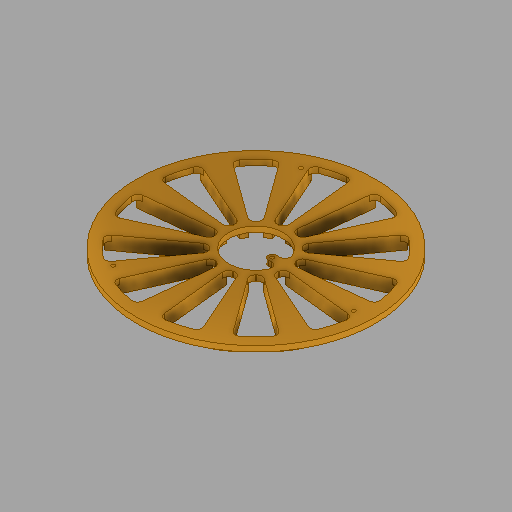
# Autodesk Inventor part: Electrode-Brass-2023-1
Saved by Autodesk Inventor 2025 (Build 290162010, 162A)
## iProperties
Created: 2021-01-06
Part Number: Electrode-Brass-2023-1
Material: Brass
Document SubType Name: Modeling
Designer: schanen
Density: 8.49 g/cm^3
Appearance: Metal 1800F Hot
Author: schanen
Autodesk Inventor part; units mm, degrees
ref_plane "YZ Plane" through (0, 0, 0) normal (1, 0, 0) x (0, 1, 0)
ref_plane "XZ Plane" through (0, 0, 0) normal (0, 1, 0) x (-1, 0, 0)
ref_plane "XY Plane" through (0, 0, 0) normal (0, 0, 1) x (1, 0, 0)
sketch "Sketch4" plane through (0, 0, 0) normal (0, 1, 0) x (-1, 0, 0)
  circle A0 centre (0, 0) radius 6 construction
  circle A1 centre (0, 0) radius 20 construction
  line L0 (0, 0) -> (-19.8904, -2.0906) construction
  line L1 (0, 0) -> (-19.8904, 2.0906) construction
  line L2 (28, 0) -> (-28, 0) projected
  arc A2 (-19.8904, 2.0906) -> (-19.8904, -2.0906) centre (0, 0) ccw
  line L3 (-19.8904, 2.0906) -> (-5.9671, 0.6272)
  line L4 (-19.8904, -2.0906) -> (-5.9671, -0.6272)
  arc A3 (-5.9671, 0.6272) -> (-5.9671, -0.6272) centre (0, 0) ccw
  dimension "d38" = 12
  dimension "d39" = 40
  dimension "d41" = 6
  dimension "d42" = 6
  constraints: 8 end point, 8 point on circle, 4 centre point, 3 coincident, 2 point on line
  measures "d38" diameter of A0
  measures "d39" diameter of A1
  measures "d41" angle of L2 L0
  measures "d42" angle of L2 L1
extrude "Extrusion5" add sketch "Sketch4" along normal blind 2.5
pattern_circular "Circular Pattern1" count 12 over 360 about axis through (0, -10, 0) along (0, 1, 0) of "Extrusion5"
sketch "Sketch5" plane through (0, 2.5, 0) normal (0, 1, 0) x (1, 0, 0)
  arc A0 (5.4813, 2.4404) -> (4.8541, 3.5267) centre (0, 0) ccw projected
  arc A1 (5.9671, -0.6272) -> (5.9671, 0.6272) centre (0, 0) ccw projected
  circle A2 centre (0, 0) radius 6
  circle A3 centre (0, 0) radius 5
  point P0 (4.8541, 3.5267)
  point P1 (5.9671, 0.6272)
  point P2 (5.4813, 2.4404)
  dimension "d48" = 1
  constraints: 2 centre point, 2 coincident, 1 concentric
  measures "d48" radial gap between concentric circles of A2 A3
extrude "Extrusion6" add sketch "Sketch5" against normal blind 1
sketch "Sketch7" plane through (0, 2.5, 0) normal (0, 1, 0) x (1, 0, 0)
  circle A0 centre (0, 0) radius 19 construction
  point P0 (18.974, -0.9944)
  point P1 (19, 0)
  dimension "d55" = 38
  dimension "d56" = -3
  constraints: 2 horizontal alignment, 1 coincident, 2 other
hole "Hole1" at (18.974, 2.5, 0.9944) direction (0, -1, 0) diameter 0.7 end through all
pattern_circular "Circular Pattern2" count 3 over 360 about axis through (0, -10, 0) along (0, 1, 0) of "Hole1"
sketch "Sketch8" plane through (0, 2.5, 0) normal (0, 1, 0) x (1, 0, 0)
  arc A0 (19.8904, -2.0906) -> (19.8904, 2.0906) centre (0, 0) ccw projected
  circle A1 centre (0, 0) radius 20
  circle A2 centre (0, 0) radius 22
  point P0 (19.8904, -2.0906)
  point P1 (19.8904, 2.0906)
  dimension "d67" = 2
  constraints: 2 centre point, 2 coincident, 1 concentric
  measures "d67" radial gap between concentric circles of A2 A1
extrude "Extrusion8" add sketch "Sketch8" against normal blind 1
fillet "Fillet5" radius 1 4 edges at (19.8904, 2, 2.0906) (19.8904, 2, -2.0906) (5.9671, 2, 0.6272) (5.9671, 2, -0.6272)
pattern_circular "Circular Pattern3" count 12 over 360 about axis through (0, 2.5, 0) along (0, -1, 0) of "Fillet5"
sketch "Sketch9" plane through (0, 2.5, 0) normal (0, 1, 0) x (1, 0, 0)
  circle A0 centre (0, 0) radius 5 projected
  line L0 (5, 0) -> (3, 0)
  line L1 (3, 0) -> (3, 0.75)
  line L2 (3, 0.75) -> (5, 0.75)
  line L3 (5, 0.75) -> (5, 0)
  line L4 (5, 0) -> (3, 0)
  line L5 (3, 0) -> (3, -0.75)
  line L6 (3, -0.75) -> (5, -0.75)
  line L7 (5, -0.75) -> (5, 0)
  circle A1 centre (3, 0) radius 0.75
  circle A2 centre (3, 0) radius 0.35
  point P0 (4.9434, -0.75)
  point P1 (4.9434, 0.75)
  dimension "d78" = 2
  dimension "d79" = 0.75
  dimension "d80" = 0.75
  dimension "d81" = 0.7
  constraints: 16 end point, 4 parallel, 2 coincident, 2 horizontal, 2 perpendicular, 1 centre point, 1 collinear, 1 horizontal alignment, 5 other
  measures "d78" distance of L1.end L2.end
  measures "d79" distance of L0.end L1.end
  measures "d80" distance of L5.end L4.end
  measures "d81" diameter of A2
extrude "Extrusion9" add sketch "Sketch9" against normal up to surface (1 mm away) contours L0 A1 L2 A0 | A0 L6 A1 L0 | A1 L5 A2 L0 | L0 A2 L1 A1 | L1 A2 L5 A1
fillet "Fillet6" radius 1 2 edges at (4.9434, 2, 0.75) (4.9434, 2, -0.75)
equation "\"d42\" = d41"
body "Solid2"
